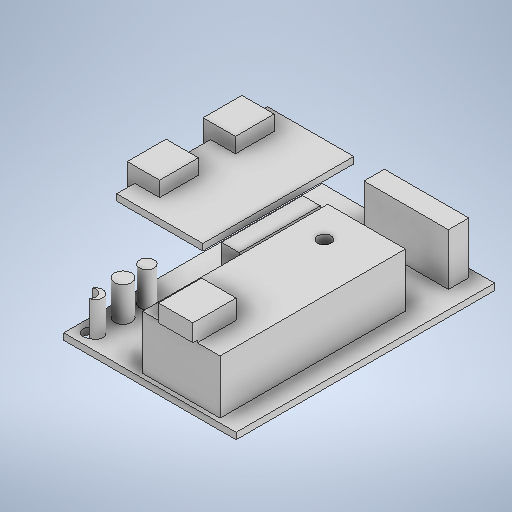
# Autodesk Inventor part: Platine
Saved by Autodesk Inventor 2025.1 (Build 291241000, 241)
## iProperties
Created: 2025-02-01
Part Number: Platine
Material: Generisch
Document SubType Name: Modeling
Designer: joebe
Density: 1 g/cm^3
Appearance: Vorgabe
Author: joebe
Autodesk Inventor part; units mm, degrees
ref_plane "YZ Plane" through (0, 0, 0) normal (1, 0, 0) x (0, 1, 0)
ref_plane "XZ Plane" through (0, 0, 0) normal (0, 1, 0) x (-1, 0, 0)
ref_plane "XY Plane" through (0, 0, 0) normal (0, 0, 1) x (1, 0, 0)
sketch "Skizze1" plane through (0, 0, 0) normal (0, 0, 1) x (1, 0, 0)
  line L0 (-20, 30) -> (20, 30)
  line L1 (20, 30) -> (20, -30)
  line L2 (20, -30) -> (-20, -30)
  line L3 (-20, -30) -> (-20, 30)
  line L4 (-20, 30) -> (20, -30) construction
  line L5 (20, 30) -> (-20, -30) construction
  point P0 (0, 0)
  dimension "d0" = 40
  dimension "d1" = 60
  constraints: 12 end point, 2 midpoint, 2 parallel, 1 horizontal, 1 perpendicular
  measures "d0" distance of L1.end L2.end
  measures "d1" distance of L0.end L1.end
extrude "Extrusion1" add sketch "Skizze1" along normal blind 1.5
sketch "Skizze2" plane through (0, 0, 1.5) normal (0, 0, 1) x (1, 0, 0)
  line L0 (-20, -30) -> (20, -30) projected
  line L1 (10, -30) -> (2, -30)
  line L2 (2, -30) -> (2, -20)
  line L3 (2, -20) -> (10, -20)
  line L4 (10, -20) -> (10, -30)
  line L5 (20, -30) -> (20, 30) projected
  point P0 (0, 0)
  dimension "d4" = 8
  dimension "d5" = 10
  dimension "d6" = 10
  constraints: 8 end point, 2 parallel, 1 horizontal, 1 perpendicular, 1 point on line
  measures "d4" distance of L2.end L3.end
  measures "d5" distance of L1.end L2.end
  measures "d6" distance between parallel lines of L5 L4
extrude "Extrusion2" add sketch "Skizze2" along normal blind 17
sketch "Skizze3" plane through (-20, -30, 0) normal (0, -1, 0) x (1, 0, 0)
  line L0 (0, 1.5) -> (22, 1.5) projected
  line L1 (30, 1.5) -> (30, 18.5) projected
  line L2 (22, 1.5) -> (30, 1.5)
  line L3 (30, 1.5) -> (30, 14.5)
  line L4 (30, 14.5) -> (22, 14.5)
  line L5 (22, 14.5) -> (22, 1.5)
  line L6 (22, 18.5) -> (30, 18.5) projected
  point P0 (20, 0)
  dimension "d9" = 4
  constraints: 8 end point, 2 parallel, 1 horizontal, 1 perpendicular, 1 point on line
  measures "d9" distance between parallel lines of L6 L4
extrude "Extrusion3" cut sketch "Skizze3" against normal blind 1
ref_plane "Arbeitsebene1" through (0, 0, 12.8) normal (0, 0, 1) x (1, 0, 0)
sketch "Skizze4" plane through (0, 0, 12.8) normal (0, 0, 1) x (1, 0, 0)
  line L0 (-29, 26.3) -> (-9, 26.3)
  line L1 (-9, 26.3) -> (-9, -8.7)
  line L2 (-9, -8.7) -> (-29, -8.7)
  line L3 (-29, -8.7) -> (-29, 26.3)
  line L4 (20, 30) -> (-20, 30) projected
  line L5 (20, -30) -> (20, 30) projected
  point P0 (0, 0)
  dimension "d12" = 35
  dimension "d13" = 20
  dimension "d14" = 3.7
  dimension "d15" = 29
  constraints: 8 end point, 2 parallel, 1 horizontal, 1 perpendicular
  measures "d12" distance of L0.end L1.end
  measures "d13" distance of L0.start L0.end
  measures "d14" distance between parallel lines of L4 L0
  measures "d15" distance between parallel lines of L1 L5
extrude "Extrusion4" add sketch "Skizze4" along normal blind 1.5
sketch "Skizze5" plane through (0, 0, 14.3) normal (0, 0, 1) x (1, 0, 0)
  line L0 (-30.75, 22.1) -> (-23.25, 22.1)
  line L1 (-23.25, 22.1) -> (-23.25, 13.1)
  line L2 (-23.25, 13.1) -> (-30.75, 13.1)
  line L3 (-30.75, 13.1) -> (-30.75, 22.1)
  line L4 (-30.75, 4.5) -> (-23.25, 4.5)
  line L5 (-23.25, 4.5) -> (-23.25, -4.5)
  line L6 (-23.25, -4.5) -> (-30.75, -4.5)
  line L7 (-30.75, -4.5) -> (-30.75, 4.5)
  line L8 (-29, 26.3) -> (-29, -8.7) projected
  line L9 (-9, 26.3) -> (-29, 26.3) projected
  line L10 (-29, -8.7) -> (-9, -8.7) projected
  point P0 (0, 0)
  dimension "d19" = 7.5
  dimension "d20" = 9
  dimension "d21" = 1.75
  dimension "d22" = 4.2
  dimension "d23" = 4.2
  dimension "d24" = 9
  constraints: 16 end point, 4 parallel, 2 horizontal, 2 perpendicular, 2 point on line
  measures "d19" distance of L0.start L0.end
  measures "d20" distance of L2.end L0.start
  measures "d21" distance between parallel lines of L8 L3
  measures "d22" distance between parallel lines of L9 L0
  measures "d23" distance between parallel lines of L10 L6
  measures "d24" distance of L6.end L4.start
extrude "Extrusion5" add sketch "Skizze5" along normal blind 3.5 and the other way blind 1.5
sketch "Skizze6" plane through (0, 0, 1.5) normal (0, 0, 1) x (1, 0, 0)
  line L0 (-2.7, -29) -> (15.3, -29)
  line L1 (15.3, -29) -> (15.3, 14)
  line L2 (15.3, 14) -> (-2.7, 14)
  line L3 (-2.7, 14) -> (-2.7, -29)
  line L4 (20, -30) -> (20, 30) projected
  point P0 (0, 0)
  point P1 (2, -29)
  dimension "d29" = 18
  dimension "d30" = 43
  dimension "d31" = 4.7
  constraints: 8 end point, 2 parallel, 1 horizontal, 1 horizontal alignment, 1 perpendicular
  measures "d29" distance of L1.end L2.end
  measures "d30" distance of L0.end L1.end
  measures "d31" distance between parallel lines of L4 L1
extrude "Extrusion6" add sketch "Skizze6" along normal blind 12.5
sketch "Skizze7" plane through (0, 0, 1.5) normal (0, 0, 1) x (1, 0, 0)
  circle A0 centre (-16.1822, -14.5102) radius 1.6858
  circle A1 centre (-16.1822, -20.0548) radius 1.97
  circle A2 centre (-16.1822, -26.455) radius 1.7027
  point P0 (0, 0)
  constraints: 3 centre point
extrude "Extrusion7" add sketch "Skizze7" along normal blind 8
sketch "Skizze8" plane through (0, 0, 1.5) normal (0, 0, 1) x (1, 0, 0)
  line L0 (-3.6658, 28.0935) -> (15.9283, 28.0935)
  line L1 (15.9283, 28.0935) -> (15.9283, 23.3572)
  line L2 (15.9283, 23.3572) -> (-3.6658, 23.3572)
  line L3 (-3.6658, 23.3572) -> (-3.6658, 28.0935)
  point P0 (0, 0)
  constraints: 8 end point, 2 parallel, 1 horizontal, 1 perpendicular
extrude "Extrusion8" add sketch "Skizze8" along normal blind 12
sketch "Skizze9" plane through (0, 0, 1.5) normal (0, 0, 1) x (1, 0, 0)
  line L0 (-7.8831, 13.3006) -> (-3.7307, 13.3006)
  line L1 (-3.7307, 13.3006) -> (-3.7307, -5.5149)
  line L2 (-3.7307, -5.5149) -> (-7.8831, -5.5149)
  line L3 (-7.8831, -5.5149) -> (-7.8831, 13.3006)
  point P0 (0, 0)
  constraints: 8 end point, 2 parallel, 1 horizontal, 1 perpendicular
extrude "Extrusion9" add sketch "Skizze9" along normal blind 12
ref_plane "Arbeitsebene2" through (0, 0, 16.25) normal (0, 0, 1) x (1, 0, 0)
sketch "Skizze10" plane through (0, 0, 16.25) normal (0, 0, 1) x (1, 0, 0)
  line L0 (-20, -30) -> (20, -30) projected
  line L1 (-20, 30) -> (-20, -30) projected
  line L2 (20, -30) -> (20, 30) projected
  point P0 (0, 0)
  point P1 (-17, -27)
  point P2 (4, 6.5)
  dimension "d40" = 3
  dimension "d41" = 3
  dimension "d42" = 16
  dimension "d43" = 36.5
  measures "d40" distance from line of point (-17, -27) L0
  measures "d41" distance from line of L1 point (-17, -27)
  measures "d42" distance from line of L2 point (4, 6.5)
  measures "d43" distance from line of L0 point (4, 6.5)
hole "Bohrung1" at (-17, -27, 16.25) at (4, 6.5, 16.25) direction (0, 0, -1) diameter 3.1 end through all
equation "\"d23\" = d22"
equation "\"d24\" = d20"
equation "\"d41\" = d40"
